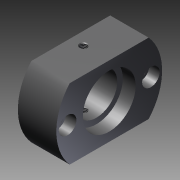
# Autodesk Inventor part: BGCSB14_h
Saved by Autodesk Inventor 2011 SP1 (Build 150282100, 282)
## iProperties
Created: 2016-11-23
Part Number: BGCSB14_h
Catalog Web Link: www.cadenas.de
Description: BGCSB, BGCS, SBGCS_housing-Bearing with Housings - Thrust Bearings - Standard
Vendor: MISUMI
Document SubType Name: Modeling
Designer: psAdmin
Manufacturer: MISUMI
Mass: 46.0645 g
Surface Area: 122.76 cm^2
Volume: 46.0645 cm^3
Density: 1 g/cm^3
Category: PARTsolutions
Company: MISUMI
Title: BGCSB14
Author: Cadenas PARTsolutions
Comments: Bearing with Housings - Thrust Bearings - Standard
PSOL_IDENT_0: {$CADENAS_DATA\23d-libs\misumi\metric\12_bearing_holders\bgcsb\housing_bgcsb.prj},184 {VTYP=3D},{NB=
PSOL_IDENT_1: BGCSB14_h},{LINA=BGCSB14},{NN=BGCSB, BGCS, SBGCS_housing},{DATE=17.06.2016 05:47:01},{GEOMDATE=02.03
PSOL_IDENT_2: .2016 00:34:00},{VERSION=},{LINEID=40},{LINESUBID=-1},{WBVAR=MAT,ST}  {NB=BGCSB14_h},{LINA=BGCSB14},
PSOL_IDENT_3: {KT=DUMMY},{PN=BGCSB14},{TYPE=BGCSB},{MAT=BG},{MAT1= 'BG','S45C Equivalent','SBG','SUS304' },{ST=B},
PSOL_IDENT_4: {ST1=    'B','Black Oxide','ENP','Electroless Nickel Plating'               },{DD=14},{D=26},{B=25},
PSOL_IDENT_5: {H=66},{W=44},{T=24},{DDZZ=17},{D1=31},{D2=33},{D3=34},{T1=16},{B1=17.0},{A=52},{F=0},{M=M8 (6.8)},{
PSOL_IDENT_6: DD1=11},{H1=6.5},{BN=NKXZ14},{DD2=6.800},{MMAX=8.000},{M1=5},{M1L=9}
NN: BGCSB, BGCS, SBGCS_housing
NT: Bearing with Housings - Thrust Bearings - Standard
NB: BGCSB14_h
NBSYN: $PN._h
LINA: BGCSB14
PN: BGCSB14
MAT: S45C Equivalent
ST: Black Oxide
DD: 14
D: 26
B: 25
H: 66
W: 44
T: 24
DDZZ: 17
D1: 31
D2: 33
D3: 34
T1: 16
B1: 17.0
A: 52
F: 0
M: M8 (6.8)
DD1: 11
H1: 6.5
BN: NKXZ14
SUPPLIER: MISUMI
ARTICLENO: BGCSB14_h
BOMINFO: BGCSB14
CREATOR: CADENAS GmbH
Autodesk Inventor part; units mm, degrees
sketch "Sketch_1" plane through (0, 0, 0) normal (0, 0, 1) x (1, 0, 0)
  line L0 (24, 0) -> (0, 0)
  line L1 (0, 33) -> (0, 13)
  line L2 (0, 13) -> (16, 13)
  line L3 (16, 13) -> (16, 16.5)
  line L4 (16, 16.5) -> (24, 16.5)
  line L5 (24, 16.5) -> (24, 33)
  line L6 (24, 33) -> (0, 33)
  constraints: 14 end point
revolve "Revolution1" add sketch "Sketch_1" angle 360 about axis through (24, 0, 0) along (1, 0, 0)
sketch "Sketch_2" plane through (0, 0, 0) normal (1, 0, 0) x (0, 1, 0)
  line L0 (-132, 88) -> (-132, -88)
  line L1 (-132, -88) -> (132, -88)
  line L2 (132, -88) -> (132, 88)
  line L3 (132, 88) -> (-132, 88)
  line L4 (-33, 22) -> (-33, -22)
  line L5 (-33, -22) -> (33, -22)
  line L6 (33, -22) -> (33, 22)
  line L7 (33, 22) -> (-33, 22)
  constraints: 16 end point
extrude "Extrusion1" cut sketch "Sketch_2" along normal blind 26
sketch "Sketch_3" plane through (0, 0, 0) normal (0, 0, 1) x (1, 0, 0)
  line L0 (24, 26) -> (0, 26)
  line L1 (0, 26) -> (0, 30)
  line L2 (0, 30) -> (0.6765, 29.3235)
  line L3 (0.6765, 29.3235) -> (16.8235, 29.3235)
  line L4 (16.8235, 29.3235) -> (17.5, 30)
  line L5 (17.5, 30) -> (17.5, 31.5)
  line L6 (17.5, 31.5) -> (24, 31.5)
  line L7 (24, 31.5) -> (24, 26)
  line L8 (24, 26) -> (0, 26)
  constraints: 18 end point
revolve "Revolution2" cut sketch "Sketch_3" angle 360 about axis through (24, 26, 0) along (1, 0, 0)
thread "Thread1" size "M8x1.25" class "6H" standard "ISO Metric profile" full length
pattern_linear "Rectangular Pattern1" count 2 spacing 52 along (0, -1, 0) of "Revolution2"
sketch "Sketch_4" plane through (8, 0, 0) normal (1, 0, 0) x (0, 0, -1)
  line L0 (-12.65, 0) -> (-22, 0)
  line L1 (-22, 0) -> (-22, 2.5)
  line L2 (-22, 2.5) -> (-21.567, 2.067)
  line L3 (-21.567, 2.067) -> (-13.083, 2.067)
  line L4 (-13.083, 2.067) -> (-12.65, 2.5)
  line L5 (-12.65, 2.5) -> (-12.65, 0)
  line L6 (-12.65, 0) -> (-22, 0)
  constraints: 14 end point
revolve "Revolution3" cut sketch "Sketch_4" angle 360 about axis through (8, 0, 12.65) along (0, 0, -1)
thread "Thread2" size "M5x0.8" class "6H" standard "ISO Metric profile" full length
sketch "Sketch_6" plane through (8, 0, 0) normal (1, 0, 0) x (0, 0, -1)
  line L0 (22, 0) -> (12.65, 0)
  line L1 (12.65, 0) -> (12.65, 2.5)
  line L2 (12.65, 2.5) -> (13.083, 2.067)
  line L3 (13.083, 2.067) -> (21.567, 2.067)
  line L4 (21.567, 2.067) -> (22, 2.5)
  line L5 (22, 2.5) -> (22, 0)
  line L6 (22, 0) -> (12.65, 0)
  constraints: 14 end point
revolve "Revolution4" cut sketch "Sketch_6" angle 360 about axis through (8, 0, -22) along (0, 0, -1)
thread "Thread3" size "M5x0.8" class "6H" standard "ISO Metric profile" full length
ref_plane "to_bearings_XY" through (16, 0, 0) normal (1, 0, 0) x (0, 0, -1)
ref_plane "to_bearings_YZ" through (16, 0, 0) normal (0, 0, -1) x (0, 1, 0)
ref_plane "to_bearings_ZX" through (16, 0, 0) normal (0, 1, 0) x (1, 0, 0)
ref_plane "to_screw1_XY" through (8, 0, 13) normal (0, 0, 1) x (1, 0, 0)
ref_plane "to_screw1_YZ" through (8, 0, 13) normal (1, 0, 0) x (0, 1, 0)
ref_plane "to_screw1_ZX" through (8, 0, 13) normal (0, 1, 0) x (0, 0, 1)
ref_plane "to_screw2_XY" through (8, 0, -13) normal (0, 0, -1) x (1, 0, 0)
ref_plane "to_screw2_YZ" through (8, 0, -13) normal (1, 0, 0) x (0, -1, 0)
ref_plane "to_screw2_ZX" through (8, 0, -13) normal (0, -1, 0) x (0, 0, -1)
body "Solid1"
